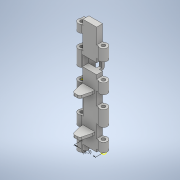
# Autodesk Inventor part: ogniwo
Saved by Autodesk Inventor 2020.3 (Build 243373000, 373)
## iProperties
Created: 2019-08-29
Part Number: ogniwo
Material: Ogólny
Document SubType Name: Modeling
Designer: patry
Density: 1 g/cm^3
Appearance: Domyślna
Author: patry
Autodesk Inventor part; units mm, degrees
ref_plane "YZ Plane" through (0, 0, 0) normal (1, 0, 0) x (0, 1, 0)
ref_plane "XZ Plane" through (0, 0, 0) normal (0, 1, 0) x (-1, 0, 0)
ref_plane "XY Plane" through (0, 0, 0) normal (0, 0, 1) x (1, 0, 0)
sketch "Szkic2" plane through (0, 0, 0) normal (0, 0, 1) x (1, 0, 0)
  circle A0 centre (0, 0) radius 1.5
  circle A1 centre (8.3, 0) radius 1.5
  circle A2 centre (0, 0) radius 0.7
  circle A3 centre (8.3, 0) radius 0.7
  dimension "d0" = 3
  dimension "d1" = 8.3
  dimension "d2" = 3
  dimension "d3" = 1.4
  dimension "d4" = 1.4
  constraints: 4 centre point, 4 coincident
  measures "d0" diameter of A0
  measures "d1" distance of point (8.3, 0) point (0, 0)
  measures "d2" diameter of A1
  measures "d3" diameter of A2
  measures "d4" diameter of A3
sketch "Szkic3" plane through (0, 0, 0) normal (0, 0, 1) x (1, 0, 0)
  line L0 (0.9267, -1.15) -> (7.3733, -1.15)
  line L1 (7.3733, -1.15) -> (7.3733, 1.15)
  line L2 (7.3733, 1.15) -> (0.9267, 1.15)
  line L3 (0.9267, 1.15) -> (0.9267, -1.15)
  line L4 (0.9267, -1.15) -> (7.3733, 1.15) construction
  line L5 (7.3733, -1.15) -> (0.9267, 1.15) construction
  point P0 (0, 0)
  point P1 (4.15, 0)
  dimension "d5" = 4.15
  dimension "d6" = 2.3
  constraints: 12 end point, 2 midpoint, 2 parallel, 1 horizontal, 1 perpendicular
  measures "d5" distance of point (0, 0) point (4.15, 0)
  measures "d6" distance of L1.end L0.end
extrude "Wyciągnięcie proste1" add sketch "Szkic2" along normal blind 45
extrude "Wyciągnięcie proste2" add sketch "Szkic3" along normal blind 45
sketch "Szkic4" plane through (0.9631, 1.15, 0) normal (0, 1, 0) x (1, 0, 0)
  line L0 (8.8369, 0) -> (8.8369, -45) projected
  line L1 (8.8369, 0) -> (8.8369, -3)
  line L2 (8.8369, -3) -> (0.5369, -3)
  line L3 (8.8369, -3) -> (5.8369, -3)
  line L4 (5.8369, -3) -> (5.8369, -4)
  line L5 (5.8369, -4) -> (8.8369, -4)
  line L6 (8.8369, -4) -> (8.8369, -3)
  line L7 (8.8369, -7.5) -> (5.8369, -7.5)
  line L8 (5.8369, -7.5) -> (5.8369, -12.5)
  line L9 (5.8369, -12.5) -> (8.8369, -12.5)
  line L10 (8.8369, -12.5) -> (8.8369, -7.5)
  line L11 (8.8369, -18.5) -> (5.8369, -18.5)
  line L12 (5.8369, -18.5) -> (5.8369, -23.5)
  line L13 (5.8369, -23.5) -> (8.8369, -23.5)
  line L14 (8.8369, -23.5) -> (8.8369, -18.5)
  line L15 (8.8369, -27.5) -> (5.8369, -27.5)
  line L16 (5.8369, -27.5) -> (5.8369, -34.5)
  line L17 (5.8369, -34.5) -> (8.8369, -34.5)
  line L18 (8.8369, -34.5) -> (8.8369, -27.5)
  line L19 (8.8369, -39) -> (5.8369, -39)
  line L20 (5.8369, -39) -> (5.8369, -45)
  line L21 (5.8369, -45) -> (8.8369, -45)
  line L22 (8.8369, -45) -> (8.8369, -39)
  line L23 (0, 0) -> (0, 0)
  line L24 (0, 0) -> (0, -45) projected
  line L25 (0, -45) -> (0, -45) projected
  line L26 (0, 0) -> (0, 0)
  line L27 (0, 0) -> (0, -45) projected
  line L28 (0, -45) -> (0, -45) projected
  line L29 (-2.4631, 0) -> (-2.4631, -45) projected
  line L30 (0, 0) -> (-2.4631, 0) projected
  line L31 (8.8369, 0) -> (6.3739, 0) projected
  line L32 (8.8369, 0) -> (0.5369, 0)
  line L33 (0.5369, 0) -> (0.5369, -3)
  line L34 (6.3739, 0) -> (0, 0) projected
  point P0 (-0.9631, 0)
  dimension "d11" = 3
  dimension "d12" = 5
  dimension "d13" = 3.5
  dimension "d14" = 1
  dimension "d15" = 5
  dimension "d16" = 6
  dimension "d17" = 7
  dimension "d18" = 4
  dimension "d19" = 4.5
  dimension "d20" = 6
  dimension "d21" = 3
  dimension "d22" = 3
  dimension "d23" = 3
  dimension "d24" = 3
  dimension "d26" = 3
  dimension "d27" = 3
  constraints: 52 end point, 10 parallel, 6 horizontal, 6 perpendicular, 6 point on line
  measures "d11" distance of L1.start L1.end
  measures "d12" distance of L8.end L7.end
  measures "d13" distance between parallel lines of L7 L5
  measures "d14" distance between parallel lines of L3 L5
  measures "d15" distance of L12.end L11.end
  measures "d16" distance between parallel lines of L9 L11
  measures "d17" distance of L16.end L15.end
  measures "d18" distance between parallel lines of L13 L15
  measures "d19" distance between parallel lines of L17 L19
  measures "d20" distance between parallel lines of L21 L19
  measures "d21" distance between parallel lines of L0 L20
  measures "d22" distance between parallel lines of L0 L16
  measures "d23" distance between parallel lines of L0 L12
  measures "d24" distance between parallel lines of L10 L8
  measures "d26" distance between parallel lines of L30 L2
  measures "d27" distance between parallel lines of L29 L33
extrude "Wyciągnięcie proste3" cut sketch "Szkic4" along normal mid plane 10
sketch "Szkic5" plane through (0.9631, 1.15, 45) normal (0, 1, 0) x (1, 0, 0)
  line L0 (6.3739, 6) -> (5.8369, 6) construction
  line L1 (0.5369, 41) -> (-2.4631, 41)
  line L2 (-2.4631, 41) -> (-2.4631, 36.5)
  line L3 (-2.4631, 36.5) -> (0.5369, 36.5)
  line L4 (0.5369, 36.5) -> (0.5369, 41)
  line L5 (0.6035, 32.5) -> (-2.4631, 32.5)
  line L6 (-2.4631, 32.5) -> (-2.4631, 25.5)
  line L7 (-2.4631, 25.5) -> (0.6035, 25.5)
  line L8 (0.6035, 25.5) -> (0.6035, 32.5)
  line L9 (0.5369, 21.5) -> (-2.4631, 21.5)
  line L10 (-2.4631, 21.5) -> (-2.4631, 16.5)
  line L11 (-2.4631, 16.5) -> (0.5369, 16.5)
  line L12 (0.5369, 16.5) -> (0.5369, 21.5)
  line L13 (0.5369, 10.5) -> (-2.4631, 10.5)
  line L14 (-2.4631, 10.5) -> (-2.4631, 5)
  line L15 (-2.4631, 5) -> (0.5369, 5)
  line L16 (0.5369, 5) -> (0.5369, 10.5)
  line L17 (0.5369, 2) -> (-2.4631, 2)
  line L18 (-2.4631, 2) -> (-2.4631, -1.3428)
  line L19 (-2.4631, -1.3428) -> (0.5369, -1.3428)
  line L20 (0.5369, -1.3428) -> (0.5369, 2)
  line L21 (6.3739, 17.5) -> (5.8369, 17.5) projected
  line L22 (5.8369, 17.5) -> (5.8369, 10.5) projected
  line L23 (5.8369, 10.5) -> (6.3739, 10.5) projected
  line L24 (6.3739, 6) -> (6.3739, 10.5) projected
  line L25 (6.3739, 6) -> (5.8369, 6) projected
  line L26 (5.8369, 6) -> (5.8369, 0) projected
  line L27 (0, 0) -> (5.8369, 0) projected
  line L28 (0, 45) -> (0, 0) projected
  line L29 (0, 45) -> (0.5369, 45) projected
  line L30 (0.5369, 45) -> (0.5369, 42) projected
  line L31 (0.5369, 42) -> (5.8369, 42) projected
  line L32 (5.8369, 42) -> (5.8369, 41) projected
  line L33 (5.8369, 41) -> (6.3739, 41) projected
  line L34 (6.3739, 37.5) -> (6.3739, 41) projected
  line L35 (6.3739, 37.5) -> (5.8369, 37.5) projected
  line L36 (5.8369, 37.5) -> (5.8369, 32.5) projected
  line L37 (5.8369, 32.5) -> (6.3739, 32.5) projected
  line L38 (6.3739, 26.5) -> (6.3739, 32.5) projected
  line L39 (6.3739, 26.5) -> (5.8369, 26.5) projected
  line L40 (5.8369, 26.5) -> (5.8369, 21.5) projected
  line L41 (5.8369, 21.5) -> (6.3739, 21.5) projected
  line L42 (6.3739, 17.5) -> (6.3739, 21.5) projected
  line L43 (5.8369, 12) -> (0.3369, 12)
  line L44 (0.3369, 12) -> (0.3369, 16)
  line L45 (0.3369, 16) -> (5.8369, 16)
  line L46 (5.8369, 16) -> (5.8369, 12)
  line L47 (-2.4631, 0) -> (0, 0) projected
  line L48 (0, 45) -> (-2.4631, 45) projected
  point P0 (-0.9631, 45)
  dimension "d32" = 3
  dimension "d33" = 5.5
  dimension "d34" = 4
  dimension "d35" = 1.5
  dimension "d78" = 5.5
  dimension "d79" = 6
  dimension "d80" = 5
  dimension "d81" = 4
  dimension "d82" = 7
  dimension "d83" = 4
  dimension "d84" = 4.5
  dimension "d85" = 2
  dimension "d86" = 4
  constraints: 48 end point, 12 parallel, 6 horizontal, 6 perpendicular, 4 point on line, 1 other
  measures "d32" distance between parallel lines of L17 L15
  measures "d33" distance of L44.end L45.end
  measures "d34" distance of L45.end L43.start
  measures "d35" distance between parallel lines of L43 L23
  measures "d78" distance between parallel lines of L15 L13
  measures "d79" distance of L13.end L10.end
  measures "d80" distance of L10.end L9.end
  measures "d81" distance of L6.end L9.end
  measures "d82" distance of L5.end L6.end
  measures "d83" distance of L2.end L5.end
  measures "d84" distance of L1.end L2.end
  measures "d85" distance from line of L17.end L47
  measures "d86" distance from line of L48 L1.end
extrude "Wyciągnięcie proste4" cut sketch "Szkic5" along normal mid plane 10 contours L4 L3 L28 L1 | L28 L3 L2 L1 | L28 L7 L6 L5 | L5 L8 L7 L28 | L28 L11 L10 L9 | L9 L12 L11 L28 | L28 L15 L14 L13 | L13 L16 L15 L28 | L28 L47 L18 L17 | L17 L20 L27 L28 | L27 L20 L19 L18 L47 | L43 L44 L45 L22
sketch "Szkic6" plane through (0, 0, 0) normal (0, 0, -1) x (-1, 0, 0)
  line L0 (-1, 1.5) -> (1.3193, 1.5) construction
  line L1 (-1.25, 1.5) -> (1.25, 1.5)
  line L2 (1.25, 1.5) -> (1.25, 4)
  line L3 (1.25, 4) -> (-1.25, 4)
  line L4 (-1.25, 4) -> (-1.25, 1.5)
  point P0 (0, 0)
  dimension "d36" = 1.5
  dimension "d37" = 2.5
  dimension "d38" = 2.5
  dimension "d39" = 1.25
  constraints: 10 end point, 2 horizontal, 2 parallel, 1 perpendicular, 1 point on line
  measures "d36" distance from line of point (0, 0) L0
  measures "d37" distance of L3.end L2.end
  measures "d38" distance of L2.end L1.end
  measures "d39" distance from line of point (0, 0) L4
extrude "Wyciągnięcie proste5" add sketch "Szkic6" against normal blind 43
chamfer "Faza1" distance 2 distance2 3.5 1 edges at (0, 4, 0) measured on face at (0, 3.5, 0)
chamfer "Faza2" distance 2 distance2 3.5 1 edges at (0, 4, 43) measured on face at (0, 3.5, 43)
sketch "Szkic7" plane through (-1.25, 1.5, 0) normal (-1, 0, 0) x (0, 0, 1)
  line L0 (39.5, 2.5) -> (43, 0.5) projected
  line L1 (3.5, 2.5) -> (39.5, 2.5) projected
  line L2 (0, 0.5) -> (3.5, 2.5) projected
  line L3 (0, 0) -> (0, 0.5) projected
  line L4 (0, 0) -> (43, 0) projected
  line L5 (43, 0.5) -> (43, 0) projected
  line L6 (0, 0) -> (4, 0) projected
  line L7 (0, -2.65) -> (0, 0) projected
  line L8 (0, -2.65) -> (4, -2.65) projected
  line L9 (4, -2.65) -> (4, 0) projected
  line L10 (4, 0) -> (4, -0.35) projected
  line L11 (4, -0.35) -> (0, -0.35) projected
  line L12 (0, 0) -> (0, -0.35) projected
  line L13 (8.5, 0) -> (12.5, 0) projected
  line L14 (8.5, 0) -> (8.5, -2.65) projected
  line L15 (8.5, -2.65) -> (12.5, -2.65) projected
  line L16 (12.5, -2.65) -> (12.5, 0) projected
  line L17 (12.5, 0) -> (12.5, -0.35) projected
  line L18 (12.5, -0.35) -> (8.5, -0.35) projected
  line L19 (8.5, -0.35) -> (8.5, 0) projected
  line L20 (19.5, 0) -> (23.5, 0) projected
  line L21 (19.5, 0) -> (19.5, -2.65) projected
  line L22 (19.5, -2.65) -> (23.5, -2.65) projected
  line L23 (23.5, -2.65) -> (23.5, 0) projected
  line L24 (23.5, 0) -> (23.5, -0.35) projected
  line L25 (23.5, -0.35) -> (19.5, -0.35) projected
  line L26 (19.5, -0.35) -> (19.5, 0) projected
  line L27 (28.5, 0) -> (34.5, 0) projected
  line L28 (28.5, 0) -> (28.5, -2.65) projected
  line L29 (28.5, -2.65) -> (34.5, -2.65) projected
  line L30 (34.5, -2.65) -> (34.5, 0) projected
  line L31 (34.5, 0) -> (34.5, -0.35) projected
  line L32 (34.5, -0.35) -> (28.5, -0.35) projected
  line L33 (28.5, -0.35) -> (28.5, 0) projected
  line L34 (40, 0) -> (43, 0) projected
  line L35 (40, 0) -> (40, -2.65) projected
  line L36 (40, -2.65) -> (43, -2.65) projected
  line L37 (43, -2.65) -> (43, 0) projected
  line L38 (43, 0) -> (43, -0.35) projected
  line L39 (43, -0.35) -> (40, -0.35) projected
  line L40 (40, -0.35) -> (40, 0) projected
  line L41 (40, -0.8) -> (43, -0.8) projected
  line L42 (43, -0.8) -> (40, -0.8)
  line L43 (40, -0.8) -> (40, 0)
  line L44 (40, 0) -> (43, 0)
  line L45 (43, 0) -> (43, -0.8)
  line L46 (34.5, -0.8) -> (28.5, -0.8)
  line L47 (28.5, -0.8) -> (28.5, 0)
  line L48 (28.5, 0) -> (34.5, 0)
  line L49 (34.5, 0) -> (34.5, -0.8)
  line L50 (23.5, -2.65) -> (23.5, -0.35) projected
  line L51 (23.5, -0.8) -> (19.5, -0.8)
  line L52 (19.5, -0.8) -> (19.5, 0)
  line L53 (19.5, 0) -> (23.5, 0)
  line L54 (23.5, 0) -> (23.5, -0.8)
  line L55 (12.5, -2.65) -> (12.5, -0.35) projected
  line L56 (12.5, -0.8) -> (8.5, -0.8)
  line L57 (8.5, -0.8) -> (8.5, 0)
  line L58 (8.5, 0) -> (12.5, 0)
  line L59 (12.5, 0) -> (12.5, -0.8)
  line L60 (0, 0) -> (43, 0) projected
  line L61 (4, -0.8) -> (0, -0.8)
  line L62 (0, -0.8) -> (0, 0)
  line L63 (0, 0) -> (4, 0)
  line L64 (4, 0) -> (4, -0.8)
  constraints: 40 end point, 10 parallel, 10 point on line, 5 horizontal, 5 perpendicular, 2 other
extrude "Wyciągnięcie proste6" add sketch "Szkic7" against normal blind 2.5 contours L37 L39 L35 L4 | L37 L41 L35 L39 | L4 L9 L11 L7 | L30 L32 L28 L4 | L11 L9 L61 L7 | L30 L46 L28 L32 | L4 L16 L18 L14 | L23 L25 L21 L4 | L18 L16 L56 L14 | L23 L51 L21 L25
ref_plane "Płaszczyzna konstrukcyjna1" through (4.5, 1.15, 34.5) normal (1, 0, 0) x (0, 0, -1)
sketch "Szkic8" plane through (4.5, 1.15, 34.5) normal (1, 0, 0) x (0, 0, -1)
  line L0 (5.5, -2.3) -> (1.5, -2.3) projected
  line L1 (5.5, -2.3) -> (5.5, 0) projected
  line L2 (1.5, 0) -> (5.5, 0) projected
  line L3 (1.5, -2.3) -> (1.5, 0) projected
  line L4 (1.5, 0) -> (5.5, 0) projected
  line L5 (1.5, 0) -> (1.5, 1)
  line L6 (1.5, 1) -> (5.5, 1)
  line L7 (5.5, 1) -> (5.5, 0)
  line L8 (5.5, 0) -> (6.5, 0)
  line L9 (6, 0) -> (0, 0) projected
  line L10 (6.5, 0) -> (6.5, 2)
  line L11 (6.5, 2) -> (0.5, 2)
  line L12 (0.5, 2) -> (0.5, 0)
  line L13 (0, 0) -> (1.5, 0) projected
  line L14 (0.5, 0) -> (1.5, 0)
  point P0 (34.5, -1.15)
  dimension "d52" = 1
  dimension "d53" = 1
  dimension "d54" = 2
  dimension "d55" = 6
  constraints: 16 end point, 6 perpendicular, 2 point on line, 1 vertical
  measures "d52" distance of L2.start L5.end
  measures "d53" distance of L1.end L8.end
  measures "d54" distance of L8.end L10.end
  measures "d55" distance of L10.end L11.end
extrude "Wyciągnięcie proste7" add sketch "Szkic8" along normal blind 1 contours L7 L6 L5 L9 L12 L11 L10 L8
fillet "Zaokrąglenie1" radius 1 2 edges at (5, 3.15, 28) (5, 3.15, 34)
sketch "Szkic9" plane through (1.5, -1.15, 3) normal (0, -1, 0) x (1, 0, 0)
  line L0 (0, 5.5) -> (4.6429, 5.5)
  line L1 (4.6429, 5.5) -> (4.6429, 6.5)
  line L2 (4.6429, 6.5) -> (0, 6.5)
  line L3 (0, 6.5) -> (0, 5.5)
  line L4 (0, 20.5) -> (4.6429, 20.5)
  line L5 (4.6429, 20.5) -> (4.6429, 19.5)
  line L6 (4.6429, 19.5) -> (0, 19.5)
  line L7 (0, 19.5) -> (0, 20.5)
  line L8 (0, 0) -> (5.3, 0) projected
  point P0 (-1.5, -3)
  dimension "d74" = 13
  dimension "d75" = 5.5
  dimension "d76" = 1
  dimension "d77" = 1
  constraints: 16 end point, 4 parallel, 2 horizontal, 2 perpendicular, 1 point on line
  measures "d74" distance between parallel lines of L2 L6
  measures "d75" distance between parallel lines of L0 L8
  measures "d76" distance of L4.end L5.end
  measures "d77" distance of L0.end L1.end
extrude "Wyciągnięcie proste8" add sketch "Szkic9" along normal blind 5
chamfer "Faza3" distance 1 distance2 4 1 edges at (1.5, -6.15, 9) measured on face at (2, -6.15, 9)
chamfer "Faza4" distance 1 distance2 4 1 edges at (1.5, -6.15, 23) measured on face at (2, -6.15, 23)
chamfer "Faza5" distance 1 distance2 4 1 edges at (6.1429, -6.15, 23) measured on face at (5.6429, -6.15, 23)
chamfer "Faza6" distance 1 distance2 4 1 edges at (6.1429, -6.15, 9) measured on face at (5.6429, -6.15, 9)
fillet "Zaokrąglenie2" radius 1 4 edges at (2.5, -6.15, 9) (5.1429, -6.15, 9) (2.5, -6.15, 23) (5.1429, -6.15, 23)
sketch "Szkic10" plane through (1.5, -1.15, 23.5) normal (0, 0, 1) x (1, 0, 0)
  point P0 (-1.5, 1.15)
sketch "Szkic11" plane through (6.8, 1.15, 3) normal (0, 0, -1) x (-1, 0, 0)
  circle A0 centre (6.8, -1.15) radius 0.7 projected
  circle A1 centre (-1.5, -1.15) radius 0.7 projected
  dimension "d87" = 8.3
  measures "d87" distance of A1.centre point (6.8, -1.15)
equation "\"d2\" = d0"
equation "\"d4\" = d3"
equation "\"d22\" = d21"
equation "\"d23\" = d22"
equation "\"d24\" = d23"
equation "\"d77\" = d76"
equation "\"dl_ogniwa\" = 9.073"
